Autodesk Fusion 360 part; units mm, degrees
(part 2 of 6)
  spline S14 degree 5 poles (-31.4433, -12.4785) (-31.4662, -12.4876) (-31.5115, -12.5064) (-31.5784, -12.5368) (-31.6657, -12.5814) (-31.7722, -12.6426) (-31.8768, -12.7077) (-31.9803, -12.7753) (-32.0831, -12.8441) (-32.1855, -12.9138) (-32.2874, -12.9845) (-32.3887, -13.0565) (-32.489, -13.1301) (-32.5883, -13.2057) (-32.6866, -13.2831) (-32.7839, -13.3623) (-32.8804, -13.443) (-32.9762, -13.5248) (-33.0713, -13.6077) (-33.1659, -13.6917) (-33.2598, -13.7766) (-33.353, -13.8626) (-33.4455, -13.9498) (-33.5373, -14.0381) (-33.6284, -14.1276) (-33.7188, -14.2182) (-33.8085, -14.3097) (-33.8976, -14.4022) (-33.986, -14.4957) (-34.0738, -14.5901) (-34.161, -14.6853) (-34.2476, -14.7815) (-34.3335, -14.8786) (-34.4188, -14.9765) (-34.5034, -15.0753) (-34.5874, -15.175) (-34.6708, -15.2756) (-34.7536, -15.3769) (-34.8357, -15.4791) (-34.9173, -15.582) (-34.9982, -15.6857) (-35.0785, -15.7902) (-35.1582, -15.8955) (-35.2373, -16.0015) (-35.3158, -16.1083) (-35.3936, -16.2158) (-35.4709, -16.324) (-35.5475, -16.433) (-35.6236, -16.5427) (-35.699, -16.653) (-35.7739, -16.764) (-35.8481, -16.8758) (-35.9218, -16.9882) (-35.9948, -17.1012) (-36.0672, -17.2149) (-36.1391, -17.3293) (-36.2103, -17.4443) (-36.2809, -17.56) (-36.351, -17.6763) (-36.4204, -17.7932) (-36.4892, -17.9107) (-36.5575, -18.0288) (-36.6251, -18.1475) (-36.6921, -18.2669) (-36.7586, -18.3868) (-36.8244, -18.5073) (-36.8897, -18.6283) (-36.9543, -18.75) (-37.0183, -18.8722) (-37.0818, -18.995) (-37.1446, -19.1183) (-37.1944, -19.2174) (-37.2315, -19.292) (-37.2561, -19.3418) (-37.2683, -19.3667) knots 0 0 0 0 0 0 0.01428571 0.02857143 0.04285714 0.05714286 0.07142857 0.08571429 0.1 0.11428571 0.12857143 0.14285714 0.15714286 0.17142857 0.18571429 0.2 0.21428571 0.22857143 0.24285714 0.25714286 0.27142857 0.28571429 0.3 0.31428571 0.32857143 0.34285714 0.35714286 0.37142857 0.38571429 0.4 0.41428571 0.42857143 0.44285714 0.45714286 0.47142857 0.48571429 0.5 0.51428571 0.52857143 0.54285714 0.55714286 0.57142857 0.58571429 0.6 0.61428571 0.62857143 0.64285714 0.65714286 0.67142857 0.68571429 0.7 0.71428571 0.72857143 0.74285714 0.75714286 0.77142857 0.78571429 0.8 0.81428571 0.82857143 0.84285714 0.85714286 0.87142857 0.88571429 0.9 0.91428571 0.92857143 0.94285714 0.95714286 0.97142857 0.98571429 1 1 1 1 1 1
  arc A30 (-37.2683, -19.3667) -> (-35.4063, -22.592) centre (0, 0) ccw
  spline S15 degree 5 poles (-35.4063, -22.592) (-35.3785, -22.5938) (-35.3231, -22.5974) (-35.2399, -22.6026) (-35.1292, -22.609) (-34.991, -22.6163) (-34.853, -22.6227) (-34.7151, -22.6284) (-34.5774, -22.6332) (-34.44, -22.6372) (-34.3027, -22.6405) (-34.1656, -22.6429) (-34.0288, -22.6445) (-33.8921, -22.6453) (-33.7557, -22.6453) (-33.6195, -22.6444) (-33.4836, -22.6427) (-33.3479, -22.6402) (-33.2124, -22.6369) (-33.0772, -22.6327) (-32.9422, -22.6277) (-32.8075, -22.6218) (-32.6731, -22.6151) (-32.5389, -22.6075) (-32.405, -22.5991) (-32.2714, -22.5898) (-32.1382, -22.5796) (-32.0052, -22.5686) (-31.8725, -22.5567) (-31.7401, -22.5439) (-31.6081, -22.5302) (-31.4764, -22.5156) (-31.345, -22.5001) (-31.214, -22.4837) (-31.0833, -22.4664) (-30.9531, -22.4482) (-30.8231, -22.4291) (-30.6936, -22.409) (-30.5644, -22.388) (-30.4357, -22.3661) (-30.3073, -22.3432) (-30.1794, -22.3193) (-30.0519, -22.2944) (-29.9249, -22.2685) (-29.7984, -22.2417) (-29.6723, -22.2138) (-29.5467, -22.1849) (-29.4215, -22.155) (-29.2968, -22.1242) (-29.1727, -22.0922) (-29.0491, -22.0592) (-28.926, -22.0251) (-28.8036, -21.9898) (-28.6819, -21.9532) (-28.5608, -21.9155) (-28.4403, -21.8767) (-28.3203, -21.8367) (-28.2009, -21.7958) (-28.0821, -21.7538) (-27.964, -21.7105) (-27.8468, -21.6658) (-27.7306, -21.6195) (-27.6155, -21.5713) (-27.5016, -21.5212) (-27.3886, -21.4695) (-27.2765, -21.4166) (-27.1649, -21.3627) (-27.0539, -21.3081) (-26.9436, -21.2522) (-26.8349, -21.1942) (-26.7287, -21.1326) (-26.6464, -21.0793) (-26.5866, -21.0365) (-26.5477, -21.0067) (-26.5284, -20.9915) knots -1 -1 -1 -1 -1 -1 -0.98571429 -0.97142857 -0.95714286 -0.94285714 -0.92857143 -0.91428571 -0.9 -0.88571429 -0.87142857 -0.85714286 -0.84285714 -0.82857143 -0.81428571 -0.8 -0.78571429 -0.77142857 -0.75714286 -0.74285714 -0.72857143 -0.71428571 -0.7 -0.68571429 -0.67142857 -0.65714286 -0.64285714 -0.62857143 -0.61428571 -0.6 -0.58571429 -0.57142857 -0.55714286 -0.54285714 -0.52857143 -0.51428571 -0.5 -0.48571429 -0.47142857 -0.45714286 -0.44285714 -0.42857143 -0.41428571 -0.4 -0.38571429 -0.37142857 -0.35714286 -0.34285714 -0.32857143 -0.31428571 -0.3 -0.28571429 -0.27142857 -0.25714286 -0.24285714 -0.22857143 -0.21428571 -0.2 -0.18571429 -0.17142857 -0.15714286 -0.14285714 -0.12857143 -0.11428571 -0.1 -0.08571429 -0.07142857 -0.05714286 -0.04285714 -0.02857143 -0.01428571 0 0 0 0 0 0
  line L15 (-26.5284, -20.9915) -> (-24.3049, -19.232)
  arc A31 (-21.5786, -19.461) -> (-24.3049, -19.232) centre (-23.0639, -20.8004) ccw
  arc A32 (-21.5786, -19.461) -> (-19.461, -21.5786) centre (0, 0) ccw
  arc A33 (-19.232, -24.3049) -> (-19.461, -21.5786) centre (-20.8004, -23.0639) ccw
  line L16 (-19.232, -24.3049) -> (-20.9915, -26.5284)
  spline S16 degree 5 poles (-20.9915, -26.5284) (-21.0067, -26.5477) (-21.0365, -26.5866) (-21.0793, -26.6464) (-21.1326, -26.7287) (-21.1942, -26.8349) (-21.2522, -26.9436) (-21.3081, -27.0539) (-21.3627, -27.1649) (-21.4166, -27.2765) (-21.4695, -27.3886) (-21.5212, -27.5016) (-21.5713, -27.6155) (-21.6195, -27.7306) (-21.6658, -27.8468) (-21.7105, -27.964) (-21.7538, -28.0821) (-21.7958, -28.2009) (-21.8367, -28.3203) (-21.8767, -28.4403) (-21.9155, -28.5608) (-21.9532, -28.6819) (-21.9898, -28.8036) (-22.0251, -28.926) (-22.0592, -29.0491) (-22.0922, -29.1727) (-22.1242, -29.2968) (-22.155, -29.4215) (-22.1849, -29.5467) (-22.2138, -29.6723) (-22.2417, -29.7984) (-22.2685, -29.9249) (-22.2944, -30.0519) (-22.3193, -30.1794) (-22.3432, -30.3073) (-22.3661, -30.4357) (-22.388, -30.5644) (-22.409, -30.6936) (-22.4291, -30.8231) (-22.4482, -30.9531) (-22.4664, -31.0833) (-22.4837, -31.214) (-22.5001, -31.345) (-22.5156, -31.4764) (-22.5302, -31.6081) (-22.5439, -31.7401) (-22.5567, -31.8725) (-22.5686, -32.0052) (-22.5796, -32.1382) (-22.5898, -32.2714) (-22.5991, -32.405) (-22.6075, -32.5389) (-22.6151, -32.6731) (-22.6218, -32.8075) (-22.6277, -32.9422) (-22.6327, -33.0772) (-22.6369, -33.2124) (-22.6402, -33.3479) (-22.6427, -33.4836) (-22.6444, -33.6195) (-22.6453, -33.7557) (-22.6453, -33.8921) (-22.6445, -34.0288) (-22.6429, -34.1656) (-22.6405, -34.3027) (-22.6372, -34.44) (-22.6332, -34.5774) (-22.6284, -34.7151) (-22.6227, -34.853) (-22.6163, -34.991) (-22.609, -35.1292) (-22.6026, -35.2399) (-22.5974, -35.3231) (-22.5938, -35.3785) (-22.592, -35.4063) knots 0 0 0 0 0 0 0.01428571 0.02857143 0.04285714 0.05714286 0.07142857 0.08571429 0.1 0.11428571 0.12857143 0.14285714 0.15714286 0.17142857 0.18571429 0.2 0.21428571 0.22857143 0.24285714 0.25714286 0.27142857 0.28571429 0.3 0.31428571 0.32857143 0.34285714 0.35714286 0.37142857 0.38571429 0.4 0.41428571 0.42857143 0.44285714 0.45714286 0.47142857 0.48571429 0.5 0.51428571 0.52857143 0.54285714 0.55714286 0.57142857 0.58571429 0.6 0.61428571 0.62857143 0.64285714 0.65714286 0.67142857 0.68571429 0.7 0.71428571 0.72857143 0.74285714 0.75714286 0.77142857 0.78571429 0.8 0.81428571 0.82857143 0.84285714 0.85714286 0.87142857 0.88571429 0.9 0.91428571 0.92857143 0.94285714 0.95714286 0.97142857 0.98571429 1 1 1 1 1 1
  arc A34 (-22.592, -35.4063) -> (-19.3667, -37.2683) centre (0, 0) ccw
  spline S17 degree 5 poles (-19.3667, -37.2683) (-19.3418, -37.2561) (-19.292, -37.2315) (-19.2174, -37.1944) (-19.1183, -37.1446) (-18.995, -37.0818) (-18.8722, -37.0183) (-18.75, -36.9543) (-18.6283, -36.8897) (-18.5073, -36.8244) (-18.3868, -36.7586) (-18.2669, -36.6921) (-18.1475, -36.6251) (-18.0288, -36.5575) (-17.9107, -36.4892) (-17.7932, -36.4204) (-17.6763, -36.351) (-17.56, -36.2809) (-17.4443, -36.2103) (-17.3293, -36.1391) (-17.2149, -36.0672) (-17.1012, -35.9948) (-16.9882, -35.9218) (-16.8758, -35.8481) (-16.764, -35.7739) (-16.653, -35.699) (-16.5427, -35.6236) (-16.433, -35.5475) (-16.324, -35.4709) (-16.2158, -35.3936) (-16.1083, -35.3158) (-16.0015, -35.2373) (-15.8955, -35.1582) (-15.7902, -35.0785) (-15.6857, -34.9982) (-15.582, -34.9173) (-15.4791, -34.8357) (-15.3769, -34.7536) (-15.2756, -34.6708) (-15.175, -34.5874) (-15.0753, -34.5034) (-14.9765, -34.4188) (-14.8786, -34.3335) (-14.7815, -34.2476) (-14.6853, -34.161) (-14.5901, -34.0738) (-14.4957, -33.986) (-14.4022, -33.8976) (-14.3097, -33.8085) (-14.2182, -33.7188) (-14.1276, -33.6284) (-14.0381, -33.5373) (-13.9498, -33.4455) (-13.8626, -33.353) (-13.7766, -33.2598) (-13.6917, -33.1659) (-13.6077, -33.0713) (-13.5248, -32.9762) (-13.443, -32.8804) (-13.3623, -32.7839) (-13.2831, -32.6866) (-13.2057, -32.5883) (-13.1301, -32.489) (-13.0565, -32.3887) (-12.9845, -32.2874) (-12.9138, -32.1855) (-12.8441, -32.0831) (-12.7753, -31.9803) (-12.7077, -31.8768) (-12.6426, -31.7722) (-12.5814, -31.6657) (-12.5368, -31.5784) (-12.5064, -31.5115) (-12.4876, -31.4662) (-12.4785, -31.4433) knots -1 -1 -1 -1 -1 -1 -0.98571429 -0.97142857 -0.95714286 -0.94285714 -0.92857143 -0.91428571 -0.9 -0.88571429 -0.87142857 -0.85714286 -0.84285714 -0.82857143 -0.81428571 -0.8 -0.78571429 -0.77142857 -0.75714286 -0.74285714 -0.72857143 -0.71428571 -0.7 -0.68571429 -0.67142857 -0.65714286 -0.64285714 -0.62857143 -0.61428571 -0.6 -0.58571429 -0.57142857 -0.55714286 -0.54285714 -0.52857143 -0.51428571 -0.5 -0.48571429 -0.47142857 -0.45714286 -0.44285714 -0.42857143 -0.41428571 -0.4 -0.38571429 -0.37142857 -0.35714286 -0.34285714 -0.32857143 -0.31428571 -0.3 -0.28571429 -0.27142857 -0.25714286 -0.24285714 -0.22857143 -0.21428571 -0.2 -0.18571429 -0.17142857 -0.15714286 -0.14285714 -0.12857143 -0.11428571 -0.1 -0.08571429 -0.07142857 -0.05714286 -0.04285714 -0.02857143 -0.01428571 0 0 0 0 0 0
  line L17 (-12.4785, -31.4433) -> (-11.4326, -28.8079)
  arc A35 (-8.9572, -27.643) -> (-11.4326, -28.8079) centre (-9.5737, -29.5456) ccw
  arc A36 (-8.9572, -27.643) -> (-6.0644, -28.4181) centre (0, 0) ccw
  arc A37 (-4.503, -30.6647) -> (-6.0644, -28.4181) centre (-6.4818, -30.3741) ccw
  line L18 (-4.503, -30.6647) -> (-4.9149, -33.47)
  spline S18 degree 5 poles (-4.9149, -33.47) (-4.9185, -33.4943) (-4.9249, -33.543) (-4.932, -33.6161) (-4.9371, -33.714) (-4.9373, -33.8368) (-4.9332, -33.96) (-4.9264, -34.0834) (-4.9182, -34.2068) (-4.9091, -34.3304) (-4.8988, -34.454) (-4.8871, -34.5776) (-4.8735, -34.7013) (-4.8577, -34.8251) (-4.8398, -34.949) (-4.8198, -35.0728) (-4.7983, -35.1967) (-4.7752, -35.3206) (-4.751, -35.4445) (-4.7256, -35.5683) (-4.699, -35.6921) (-4.6711, -35.8159) (-4.6419, -35.9396) (-4.6113, -36.0632) (-4.5793, -36.1868) (-4.5461, -36.3104) (-4.5117, -36.4339) (-4.4761, -36.5573) (-4.4394, -36.6806) (-4.4016, -36.8038) (-4.3627, -36.927) (-4.3226, -37.05) (-4.2815, -37.173) (-4.2393, -37.2958) (-4.1961, -37.4185) (-4.1517, -37.5411) (-4.1064, -37.6636) (-4.06, -37.7859) (-4.0126, -37.9082) (-3.9642, -38.0302) (-3.9148, -38.1522) (-3.8645, -38.274) (-3.8132, -38.3956) (-3.7609, -38.5172) (-3.7077, -38.6385) (-3.6535, -38.7597) (-3.5984, -38.8807) (-3.5424, -39.0016) (-3.4854, -39.1223) (-3.4276, -39.2428) (-3.3689, -39.3631) (-3.3092, -39.4833) (-3.2487, -39.6032) (-3.1873, -39.723) (-3.125, -39.8426) (-3.0619, -39.962) (-2.9979, -40.0812) (-2.9331, -40.2002) (-2.8674, -40.319) (-2.8009, -40.4376) (-2.7335, -40.5559) (-2.6653, -40.6741) (-2.5963, -40.792) (-2.5265, -40.9098) (-2.4559, -41.0273) (-2.3844, -41.1445) (-2.3122, -41.2616) (-2.2392, -41.3783) (-2.1654, -41.4949) (-2.0908, -41.6112) (-2.0154, -41.7273) (-1.9545, -41.82) (-1.9084, -41.8894) (-1.8776, -41.9356) (-1.8621, -41.9587) knots 0 0 0 0 0 0 0.01428571 0.02857143 0.04285714 0.05714286 0.07142857 0.08571429 0.1 0.11428571 0.12857143 0.14285714 0.15714286 0.17142857 0.18571429 0.2 0.21428571 0.22857143 0.24285714 0.25714286 0.27142857 0.28571429 0.3 0.31428571 0.32857143 0.34285714 0.35714286 0.37142857 0.38571429 0.4 0.41428571 0.42857143 0.44285714 0.45714286 0.47142857 0.48571429 0.5 0.51428571 0.52857143 0.54285714 0.55714286 0.57142857 0.58571429 0.6 0.61428571 0.62857143 0.64285714 0.65714286 0.67142857 0.68571429 0.7 0.71428571 0.72857143 0.74285714 0.75714286 0.77142857 0.78571429 0.8 0.81428571 0.82857143 0.84285714 0.85714286 0.87142857 0.88571429 0.9 0.91428571 0.92857143 0.94285714 0.95714286 0.97142857 0.98571429 1 1 1 1 1 1
  arc A38 (-1.8621, -41.9587) -> (1.8621, -41.9587) centre (0, 0) ccw
  spline S19 degree 5 poles (1.8621, -41.9587) (1.8776, -41.9356) (1.9084, -41.8894) (1.9545, -41.82) (2.0154, -41.7273) (2.0908, -41.6112) (2.1654, -41.4949) (2.2392, -41.3783) (2.3122, -41.2616) (2.3844, -41.1445) (2.4559, -41.0273) (2.5265, -40.9098) (2.5963, -40.792) (2.6653, -40.6741) (2.7335, -40.5559) (2.8009, -40.4376) (2.8674, -40.319) (2.9331, -40.2002) (2.9979, -40.0812) (3.0619, -39.962) (3.125, -39.8426) (3.1873, -39.723) (3.2487, -39.6032) (3.3092, -39.4833) (3.3689, -39.3631) (3.4276, -39.2428) (3.4854, -39.1223) (3.5424, -39.0016) (3.5984, -38.8807) (3.6535, -38.7597) (3.7077, -38.6385) (3.7609, -38.5172) (3.8132, -38.3956) (3.8645, -38.274) (3.9148, -38.1522) (3.9642, -38.0302) (4.0126, -37.9082) (4.06, -37.7859) (4.1064, -37.6636) (4.1517, -37.5411) (4.1961, -37.4185) (4.2393, -37.2958) (4.2815, -37.173) (4.3226, -37.05) (4.3627, -36.927) (4.4016, -36.8038) (4.4394, -36.6806) (4.4761, -36.5573) (4.5117, -36.4339) (4.5461, -36.3104) (4.5793, -36.1868) (4.6113, -36.0632) (4.6419, -35.9396) (4.6711, -35.8159) (4.699, -35.6921) (4.7256, -35.5683) (4.751, -35.4445) (4.7752, -35.3206) (4.7983, -35.1967) (4.8198, -35.0728) (4.8398, -34.949) (4.8577, -34.8251) (4.8735, -34.7013) (4.8871, -34.5776) (4.8988, -34.454) (4.9091, -34.3304) (4.9182, -34.2068) (4.9264, -34.0834) (4.9332, -33.96) (4.9373, -33.8368) (4.9371, -33.714) (4.932, -33.6161) (4.9249, -33.543) (4.9185, -33.4943) (4.9149, -33.47) knots -1 -1 -1 -1 -1 -1 -0.98571429 -0.97142857 -0.95714286 -0.94285714 -0.92857143 -0.91428571 -0.9 -0.88571429 -0.87142857 -0.85714286 -0.84285714 -0.82857143 -0.81428571 -0.8 -0.78571429 -0.77142857 -0.75714286 -0.74285714 -0.72857143 -0.71428571 -0.7 -0.68571429 -0.67142857 -0.65714286 -0.64285714 -0.62857143 -0.61428571 -0.6 -0.58571429 -0.57142857 -0.55714286 -0.54285714 -0.52857143 -0.51428571 -0.5 -0.48571429 -0.47142857 -0.45714286 -0.44285714 -0.42857143 -0.41428571 -0.4 -0.38571429 -0.37142857 -0.35714286 -0.34285714 -0.32857143 -0.31428571 -0.3 -0.28571429 -0.27142857 -0.25714286 -0.24285714 -0.22857143 -0.21428571 -0.2 -0.18571429 -0.17142857 -0.15714286 -0.14285714 -0.12857143 -0.11428571 -0.1 -0.08571429 -0.07142857 -0.05714286 -0.04285714 -0.02857143 -0.01428571 0 0 0 0 0 0
  line L19 (4.9149, -33.47) -> (4.503, -30.6647)
  arc A39 (6.0644, -28.4181) -> (4.503, -30.6647) centre (6.4818, -30.3741) ccw
  arc A40 (6.0644, -28.4181) -> (8.9572, -27.643) centre (0, 0) ccw
  arc A41 (11.4326, -28.8079) -> (8.9572, -27.643) centre (9.5737, -29.5456) ccw
  line L20 (11.4326, -28.8079) -> (12.4785, -31.4433)
  spline S20 degree 5 poles (12.4785, -31.4433) (12.4876, -31.4662) (12.5064, -31.5115) (12.5368, -31.5784) (12.5814, -31.6657) (12.6426, -31.7722) (12.7077, -31.8768) (12.7753, -31.9803) (12.8441, -32.0831) (12.9138, -32.1855) (12.9845, -32.2874) (13.0565, -32.3887) (13.1301, -32.489) (13.2057, -32.5883) (13.2831, -32.6866) (13.3623, -32.7839) (13.443, -32.8804) (13.5248, -32.9762) (13.6077, -33.0713) (13.6917, -33.1659) (13.7766, -33.2598) (13.8626, -33.353) (13.9498, -33.4455) (14.0381, -33.5373) (14.1276, -33.6284) (14.2182, -33.7188) (14.3097, -33.8085) (14.4022, -33.8976) (14.4957, -33.986) (14.5901, -34.0738) (14.6853, -34.161) (14.7815, -34.2476) (14.8786, -34.3335) (14.9765, -34.4188) (15.0753, -34.5034) (15.175, -34.5874) (15.2756, -34.6708) (15.3769, -34.7536) (15.4791, -34.8357) (15.582, -34.9173) (15.6857, -34.9982) (15.7902, -35.0785) (15.8955, -35.1582) (16.0015, -35.2373) (16.1083, -35.3158) (16.2158, -35.3936) (16.324, -35.4709) (16.433, -35.5475) (16.5427, -35.6236) (16.653, -35.699) (16.764, -35.7739) (16.8758, -35.8481) (16.9882, -35.9218) (17.1012, -35.9948) (17.2149, -36.0672) (17.3293, -36.1391) (17.4443, -36.2103) (17.56, -36.2809) (17.6763, -36.351) (17.7932, -36.4204) (17.9107, -36.4892) (18.0288, -36.5575) (18.1475, -36.6251) (18.2669, -36.6921) (18.3868, -36.7586) (18.5073, -36.8244) (18.6283, -36.8897) (18.75, -36.9543) (18.8722, -37.0183) (18.995, -37.0818) (19.1183, -37.1446) (19.2174, -37.1944) (19.292, -37.2315) (19.3418, -37.2561) (19.3667, -37.2683) knots 0 0 0 0 0 0 0.01428571 0.02857143 0.04285714 0.05714286 0.07142857 0.08571429 0.1 0.11428571 0.12857143 0.14285714 0.15714286 0.17142857 0.18571429 0.2 0.21428571 0.22857143 0.24285714 0.25714286 0.27142857 0.28571429 0.3 0.31428571 0.32857143 0.34285714 0.35714286 0.37142857 0.38571429 0.4 0.41428571 0.42857143 0.44285714 0.45714286 0.47142857 0.48571429 0.5 0.51428571 0.52857143 0.54285714 0.55714286 0.57142857 0.58571429 0.6 0.61428571 0.62857143 0.64285714 0.65714286 0.67142857 0.68571429 0.7 0.71428571 0.72857143 0.74285714 0.75714286 0.77142857 0.78571429 0.8 0.81428571 0.82857143 0.84285714 0.85714286 0.87142857 0.88571429 0.9 0.91428571 0.92857143 0.94285714 0.95714286 0.97142857 0.98571429 1 1 1 1 1 1
  arc A42 (19.3667, -37.2683) -> (22.592, -35.4063) centre (0, 0) ccw
  spline S21 degree 5 poles (22.592, -35.4063) (22.5938, -35.3785) (22.5974, -35.3231) (22.6026, -35.2399) (22.609, -35.1292) (22.6163, -34.991) (22.6227, -34.853) (22.6284, -34.7151) (22.6332, -34.5774) (22.6372, -34.44) (22.6405, -34.3027) (22.6429, -34.1656) (22.6445, -34.0288) (22.6453, -33.8921) (22.6453, -33.7557) (22.6444, -33.6195) (22.6427, -33.4836) (22.6402, -33.3479) (22.6369, -33.2124) (22.6327, -33.0772) (22.6277, -32.9422) (22.6218, -32.8075) (22.6151, -32.6731) (22.6075, -32.5389) (22.5991, -32.405) (22.5898, -32.2714) (22.5796, -32.1382) (22.5686, -32.0052) (22.5567, -31.8725) (22.5439, -31.7401) (22.5302, -31.6081) (22.5156, -31.4764) (22.5001, -31.345) (22.4837, -31.214) (22.4664, -31.0833) (22.4482, -30.9531) (22.4291, -30.8231) (22.409, -30.6936) (22.388, -30.5644) (22.3661, -30.4357) (22.3432, -30.3073) (22.3193, -30.1794) (22.2944, -30.0519) (22.2685, -29.9249) (22.2417, -29.7984) (22.2138, -29.6723) (22.1849, -29.5467) (22.155, -29.4215) (22.1242, -29.2968) (22.0922, -29.1727) (22.0592, -29.0491) (22.0251, -28.926) (21.9898, -28.8036) (21.9532, -28.6819) (21.9155, -28.5608) (21.8767, -28.4403) (21.8367, -28.3203) (21.7958, -28.2009) (21.7538, -28.0821) (21.7105, -27.964) (21.6658, -27.8468) (21.6195, -27.7306) (21.5713, -27.6155) (21.5212, -27.5016) (21.4695, -27.3886) (21.4166, -27.2765) (21.3627, -27.1649) (21.3081, -27.0539) (21.2522, -26.9436) (21.1942, -26.8349) (21.1326, -26.7287) (21.0793, -26.6464) (21.0365, -26.5866) (21.0067, -26.5477) (20.9915, -26.5284) knots -1 -1 -1 -1 -1 -1 -0.98571429 -0.97142857 -0.95714286 -0.94285714 -0.92857143 -0.91428571 -0.9 -0.88571429 -0.87142857 -0.85714286 -0.84285714 -0.82857143 -0.81428571 -0.8 -0.78571429 -0.77142857 -0.75714286 -0.74285714 -0.72857143 -0.71428571 -0.7 -0.68571429 -0.67142857 -0.65714286 -0.64285714 -0.62857143 -0.61428571 -0.6 -0.58571429 -0.57142857 -0.55714286 -0.54285714 -0.52857143 -0.51428571 -0.5 -0.48571429 -0.47142857 -0.45714286 -0.44285714 -0.42857143 -0.41428571 -0.4 -0.38571429 -0.37142857 -0.35714286 -0.34285714 -0.32857143 -0.31428571 -0.3 -0.28571429 -0.27142857 -0.25714286 -0.24285714 -0.22857143 -0.21428571 -0.2 -0.18571429 -0.17142857 -0.15714286 -0.14285714 -0.12857143 -0.11428571 -0.1 -0.08571429 -0.07142857 -0.05714286 -0.04285714 -0.02857143 -0.01428571 0 0 0 0 0 0
  line L21 (20.9915, -26.5284) -> (19.232, -24.3049)
  arc A43 (19.461, -21.5786) -> (19.232, -24.3049) centre (20.8004, -23.0639) ccw
  arc A44 (19.461, -21.5786) -> (21.5786, -19.461) centre (0, 0) ccw
  arc A45 (24.3049, -19.232) -> (21.5786, -19.461) centre (23.0639, -20.8004) ccw
  line L22 (24.3049, -19.232) -> (26.5284, -20.9915)
  spline S22 degree 5 poles (26.5284, -20.9915) (26.5477, -21.0067) (26.5866, -21.0365) (26.6464, -21.0793) (26.7287, -21.1326) (26.8349, -21.1942) (26.9436, -21.2522) (27.0539, -21.3081) (27.1649, -21.3627) (27.2765, -21.4166) (27.3886, -21.4695) (27.5016, -21.5212) (27.6155, -21.5713) (27.7306, -21.6195) (27.8468, -21.6658) (27.964, -21.7105) (28.0821, -21.7538) (28.2009, -21.7958) (28.3203, -21.8367) (28.4403, -21.8767) (28.5608, -21.9155) (28.6819, -21.9532) (28.8036, -21.9898) (28.926, -22.0251) (29.0491, -22.0592) (29.1727, -22.0922) (29.2968, -22.1242) (29.4215, -22.155) (29.5467, -22.1849) (29.6723, -22.2138) (29.7984, -22.2417) (29.9249, -22.2685) (30.0519, -22.2944) (30.1794, -22.3193) (30.3073, -22.3432) (30.4357, -22.3661) (30.5644, -22.388) (30.6936, -22.409) (30.8231, -22.4291) (30.9531, -22.4482) (31.0833, -22.4664) (31.214, -22.4837) (31.345, -22.5001) (31.4764, -22.5156) (31.6081, -22.5302) (31.7401, -22.5439) (31.8725, -22.5567) (32.0052, -22.5686) (32.1382, -22.5796) (32.2714, -22.5898) (32.405, -22.5991) (32.5389, -22.6075) (32.6731, -22.6151) (32.8075, -22.6218) (32.9422, -22.6277) (33.0772, -22.6327) (33.2124, -22.6369) (33.3479, -22.6402) (33.4836, -22.6427) (33.6195, -22.6444) (33.7557, -22.6453) (33.8921, -22.6453) (34.0288, -22.6445) (34.1656, -22.6429) (34.3027, -22.6405) (34.44, -22.6372) (34.5774, -22.6332) (34.7151, -22.6284) (34.853, -22.6227) (34.991, -22.6163) (35.1292, -22.609) (35.2399, -22.6026) (35.3231, -22.5974) (35.3785, -22.5938) (35.4063, -22.592) knots 0 0 0 0 0 0 0.01428571 0.02857143 0.04285714 0.05714286 0.07142857 0.08571429 0.1 0.11428571 0.12857143 0.14285714 0.15714286 0.17142857 0.18571429 0.2 0.21428571 0.22857143 0.24285714 0.25714286 0.27142857 0.28571429 0.3 0.31428571 0.32857143 0.34285714 0.35714286 0.37142857 0.38571429 0.4 0.41428571 0.42857143 0.44285714 0.45714286 0.47142857 0.48571429 0.5 0.51428571 0.52857143 0.54285714 0.55714286 0.57142857 0.58571429 0.6 0.61428571 0.62857143 0.64285714 0.65714286 0.67142857 0.68571429 0.7 0.71428571 0.72857143 0.74285714 0.75714286 0.77142857 0.78571429 0.8 0.81428571 0.82857143 0.84285714 0.85714286 0.87142857 0.88571429 0.9 0.91428571 0.92857143 0.94285714 0.95714286 0.97142857 0.98571429 1 1 1 1 1 1
  arc A46 (35.4063, -22.592) -> (37.2683, -19.3667) centre (0, 0) ccw
  spline S23 degree 5 poles (37.2683, -19.3667) (37.2561, -19.3418) (37.2315, -19.292) (37.1944, -19.2174) (37.1446, -19.1183) (37.0818, -18.995) (37.0183, -18.8722) (36.9543, -18.75) (36.8897, -18.6283) (36.8244, -18.5073) (36.7586, -18.3868) (36.6921, -18.2669) (36.6251, -18.1475) (36.5575, -18.0288) (36.4892, -17.9107) (36.4204, -17.7932) (36.351, -17.6763) (36.2809, -17.56) (36.2103, -17.4443) (36.1391, -17.3293) (36.0672, -17.2149) (35.9948, -17.1012) (35.9218, -16.9882) (35.8481, -16.8758) (35.7739, -16.764) (35.699, -16.653) (35.6236, -16.5427) (35.5475, -16.433) (35.4709, -16.324) (35.3936, -16.2158) (35.3158, -16.1083) (35.2373, -16.0015) (35.1582, -15.8955) (35.0785, -15.7902) (34.9982, -15.6857) (34.9173, -15.582) (34.8357, -15.4791) (34.7536, -15.3769) (34.6708, -15.2756) (34.5874, -15.175) (34.5034, -15.0753) (34.4188, -14.9765) (34.3335, -14.8786) (34.2476, -14.7815) (34.161, -14.6853) (34.0738, -14.5901) (33.986, -14.4957) (33.8976, -14.4022) (33.8085, -14.3097) (33.7188, -14.2182) (33.6284, -14.1276) (33.5373, -14.0381) (33.4455, -13.9498) (33.353, -13.8626) (33.2598, -13.7766) (33.1659, -13.6917) (33.0713, -13.6077) (32.9762, -13.5248) (32.8804, -13.443) (32.7839, -13.3623) (32.6866, -13.2831) (32.5883, -13.2057) (32.489, -13.1301) (32.3887, -13.0565) (32.2874, -12.9845) (32.1855, -12.9138) (32.0831, -12.8441) (31.9803, -12.7753) (31.8768, -12.7077) (31.7722, -12.6426) (31.6657, -12.5814) (31.5784, -12.5368) (31.5115, -12.5064) (31.4662, -12.4876) (31.4433, -12.4785) knots -1 -1 -1 -1 -1 -1 -0.98571429 -0.97142857 -0.95714286 -0.94285714 -0.92857143 -0.91428571 -0.9 -0.88571429 -0.87142857 -0.85714286 -0.84285714 -0.82857143 -0.81428571 -0.8 -0.78571429 -0.77142857 -0.75714286 -0.74285714 -0.72857143 -0.71428571 -0.7 -0.68571429 -0.67142857 -0.65714286 -0.64285714 -0.62857143 -0.61428571 -0.6 -0.58571429 -0.57142857 -0.55714286 -0.54285714 -0.52857143 -0.51428571 -0.5 -0.48571429 -0.47142857 -0.45714286 -0.44285714 -0.42857143 -0.41428571 -0.4 -0.38571429 -0.37142857 -0.35714286 -0.34285714 -0.32857143 -0.31428571 -0.3 -0.28571429 -0.27142857 -0.25714286 -0.24285714 -0.22857143 -0.21428571 -0.2 -0.18571429 -0.17142857 -0.15714286 -0.14285714 -0.12857143 -0.11428571 -0.1 -0.08571429 -0.07142857 -0.05714286 -0.04285714 -0.02857143 -0.01428571 0 0 0 0 0 0
  line L23 (31.4433, -12.4785) -> (28.8079, -11.4326)
  arc A47 (27.643, -8.9572) -> (28.8079, -11.4326) centre (29.5456, -9.5737) ccw
  circle A48 centre (0, 0) radius 2.5
  arc A49 (173.4789, -18.1364) -> (174.1765, -15.5329) centre (111, 0) ccw
  arc A50 (176.538, -14.0549) -> (174.1765, -15.5329) centre (176.1187, -16.0104) ccw
  line L24 (176.538, -14.0549) -> (177.1537, -14.1869)
  spline S24 degree 5 poles (177.1537, -14.1869) (177.1836, -14.1933) (177.2435, -14.2054) (177.3338, -14.2212) (177.4547, -14.2379) (177.6068, -14.2529) (177.7596, -14.2636) (177.9128, -14.2716) (178.0662, -14.2783) (178.2197, -14.284) (178.3734, -14.2887) (178.5272, -14.2921) (178.6813, -14.2937) (178.8356, -14.2932) (178.9902, -14.2907) (179.145, -14.2862) (179.2999, -14.2801) (179.455, -14.2726) (179.6102, -14.2639) (179.7655, -14.2541) (179.9208, -14.2432) (180.0763, -14.231) (180.2318, -14.2177) (180.3875, -14.203) (180.5432, -14.187) (180.699, -14.1699) (180.8549, -14.1515) (181.0108, -14.1321) (181.1668, -14.1116) (181.3228, -14.0901) (181.4789, -14.0675) (181.635, -14.0439) (181.7911, -14.0193) (181.9473, -13.9936) (182.1034, -13.9669) (182.2596, -13.9393) (182.4159, -13.9106) (182.5721, -13.881) (182.7284, -13.8504) (182.8846, -13.8189) (183.0409, -13.7865) (183.1971, -13.7532) (183.3533, -13.7189) (183.5096, -13.6838) (183.6658, -13.6477) (183.822, -13.6108) (183.9782, -13.573) (184.1343, -13.5344) (184.2905, -13.4948) (184.4466, -13.4545) (184.6026, -13.4132) (184.7587, -13.3712) (184.9147, -13.3283) (185.0707, -13.2846) (185.2266, -13.2401) (185.3825, -13.1947) (185.5383, -13.1486) (185.6941, -13.1017) (185.8498, -13.0539) (186.0055, -13.0054) (186.1611, -12.9561) (186.3167, -12.9061) (186.4722, -12.8552) (186.6276, -12.8036) (186.783, -12.7512) (186.9383, -12.6981) (187.0935, -12.6442) (187.2487, -12.5896) (187.4037, -12.5342) (187.5587, -12.4781) (187.7137, -12.4213) (187.8375, -12.3752) (187.9304, -12.3403) (187.9923, -12.3169) (188.0233, -12.3052) knots 0 0 0 0 0 0 0.01428571 0.02857143 0.04285714 0.05714286 0.07142857 0.08571429 0.1 0.11428571 0.12857143 0.14285714 0.15714286 0.17142857 0.18571429 0.2 0.21428571 0.22857143 0.24285714 0.25714286 0.27142857 0.28571429 0.3 0.31428571 0.32857143 0.34285714 0.35714286 0.37142857 0.38571429 0.4 0.41428571 0.42857143 0.44285714 0.45714286 0.47142857 0.48571429 0.5 0.51428571 0.52857143 0.54285714 0.55714286 0.57142857 0.58571429 0.6 0.61428571 0.62857143 0.64285714 0.65714286 0.67142857 0.68571429 0.7 0.71428571 0.72857143 0.74285714 0.75714286 0.77142857 0.78571429 0.8 0.81428571 0.82857143 0.84285714 0.85714286 0.87142857 0.88571429 0.9 0.91428571 0.92857143 0.94285714 0.95714286 0.97142857 0.98571429 1 1 1 1 1 1
  arc A51 (188.0233, -12.3052) -> (188.5836, -8.0492) centre (111, 0) ccw
  spline S25 degree 5 poles (188.5836, -8.0492) (188.5567, -8.0298) (188.503, -7.9912) (188.4223, -7.9335) (188.3146, -7.8569) (188.1796, -7.7619) (188.0444, -7.6676) (187.909, -7.574) (187.7732, -7.4811) (187.6373, -7.3889) (187.501, -7.2973) (187.3645, -7.2065) (187.2277, -7.1165) (187.0906, -7.0271) (186.9533, -6.9385) (186.8158, -6.8506) (186.678, -6.7634) (186.5399, -6.677) (186.4016, -6.5913) (186.263, -6.5065) (186.1242, -6.4223) (185.9851, -6.339) (185.8457, -6.2564) (185.7061, -6.1746) (185.5663, -6.0936) (185.4262, -6.0134) (185.2859, -5.934) (185.1453, -5.8554) (185.0045, -5.7776) (184.8634, -5.7007) (184.7221, -5.6246) (184.5805, -5.5493) (184.4387, -5.4749) (184.2966, -5.4014) (184.1543, -5.3288) (184.0118, -5.257) (183.869, -5.1862) (183.726, -5.1162) (183.5828, -5.0472) (183.4393, -4.9791) (183.2956, -4.9119) (183.1516, -4.8457) (183.0074, -4.7805) (182.863, -4.7163) (182.7183, -4.6531) (182.5734, -4.5909) (182.4283, -4.5297) (182.2829, -4.4696) (182.1373, -4.4104) (181.9915, -4.3524) (181.8454, -4.2955) (181.6991, -4.2398) (181.5526, -4.1853) (181.4058, -4.1321) (181.2588, -4.0802) (181.1116, -4.0294) (180.9641, -3.9798) (180.8165, -3.9312) (180.6686, -3.8838) (180.5205, -3.8378) (180.3722, -3.7934) (180.2235, -3.751) (180.0746, -3.7106) (179.9254, -3.6722) (179.7759, -3.6356) (179.6262, -3.6004) (179.4764, -3.5662) (179.3265, -3.533) (179.1765, -3.5011) (179.0261, -3.4719) (178.8753, -3.447) (178.7542, -3.4318) (178.663, -3.4237) (178.602, -3.4199) (178.5715, -3.4183) knots -1 -1 -1 -1 -1 -1 -0.98571429 -0.97142857 -0.95714286 -0.94285714 -0.92857143 -0.91428571 -0.9 -0.88571429 -0.87142857 -0.85714286 -0.84285714 -0.82857143 -0.81428571 -0.8 -0.78571429 -0.77142857 -0.75714286 -0.74285714 -0.72857143 -0.71428571 -0.7 -0.68571429 -0.67142857 -0.65714286 -0.64285714 -0.62857143 -0.61428571 -0.6 -0.58571429 -0.57142857 -0.55714286 -0.54285714 -0.52857143 -0.51428571 -0.5 -0.48571429 -0.47142857 -0.45714286 -0.44285714 -0.42857143 -0.41428571 -0.4 -0.38571429 -0.37142857 -0.35714286 -0.34285714 -0.32857143 -0.31428571 -0.3 -0.28571429 -0.27142857 -0.25714286 -0.24285714 -0.22857143 -0.21428571 -0.2 -0.18571429 -0.17142857 -0.15714286 -0.14285714 -0.12857143 -0.11428571 -0.1 -0.08571429 -0.07142857 -0.05714286 -0.04285714 -0.02857143 -0.01428571 0 0 0 0 0 0
  line L25 (178.5715, -3.4183) -> (177.9426, -3.3865)
  arc A52 (176.044, -1.3477) -> (177.9426, -3.3865) centre (178.0436, -1.3891) ccw
  arc A53 (176.044, -1.3477) -> (176.044, 1.3477) centre (111, 0) ccw
  arc A54 (177.9426, 3.3865) -> (176.044, 1.3477) centre (178.0436, 1.3891) ccw
  line L26 (177.9426, 3.3865) -> (178.5715, 3.4183)
  spline S26 degree 5 poles (178.5715, 3.4183) (178.602, 3.4199) (178.663, 3.4237) (178.7542, 3.4318) (178.8753, 3.447) (179.0261, 3.4719) (179.1765, 3.5011) (179.3265, 3.533) (179.4764, 3.5662) (179.6262, 3.6004) (179.7759, 3.6356) (179.9254, 3.6722) (180.0746, 3.7106) (180.2235, 3.751) (180.3722, 3.7934) (180.5205, 3.8378) (180.6686, 3.8838) (180.8165, 3.9312) (180.9641, 3.9798) (181.1116, 4.0294) (181.2588, 4.0802) (181.4058, 4.1321) (181.5526, 4.1853) (181.6991, 4.2398) (181.8454, 4.2955) (181.9915, 4.3524) (182.1373, 4.4104) (182.2829, 4.4696) (182.4283, 4.5297) (182.5734, 4.5909) (182.7183, 4.6531) (182.863, 4.7163) (183.0074, 4.7805) (183.1516, 4.8457) (183.2956, 4.9119) (183.4393, 4.9791) (183.5828, 5.0472) (183.726, 5.1162) (183.869, 5.1862) (184.0118, 5.257) (184.1543, 5.3288) (184.2966, 5.4014) (184.4387, 5.4749) (184.5805, 5.5493) (184.7221, 5.6246) (184.8634, 5.7007) (185.0045, 5.7776) (185.1453, 5.8554) (185.2859, 5.934) (185.4262, 6.0134) (185.5663, 6.0936) (185.7061, 6.1746) (185.8457, 6.2564) (185.9851, 6.339) (186.1242, 6.4223) (186.263, 6.5065) (186.4016, 6.5913) (186.5399, 6.677) (186.678, 6.7634) (186.8158, 6.8506) (186.9533, 6.9385) (187.0906, 7.0271) (187.2277, 7.1165) (187.3645, 7.2065) (187.501, 7.2973) (187.6373, 7.3889) (187.7732, 7.4811) (187.909, 7.574) (188.0444, 7.6676) (188.1796, 7.7619) (188.3146, 7.8569) (188.4223, 7.9335) (188.503, 7.9912) (188.5567, 8.0298) (188.5836, 8.0492) knots 0 0 0 0 0 0 0.01428571 0.02857143 0.04285714 0.05714286 0.07142857 0.08571429 0.1 0.11428571 0.12857143 0.14285714 0.15714286 0.17142857 0.18571429 0.2 0.21428571 0.22857143 0.24285714 0.25714286 0.27142857 0.28571429 0.3 0.31428571 0.32857143 0.34285714 0.35714286 0.37142857 0.38571429 0.4 0.41428571 0.42857143 0.44285714 0.45714286 0.47142857 0.48571429 0.5 0.51428571 0.52857143 0.54285714 0.55714286 0.57142857 0.58571429 0.6 0.61428571 0.62857143 0.64285714 0.65714286 0.67142857 0.68571429 0.7 0.71428571 0.72857143 0.74285714 0.75714286 0.77142857 0.78571429 0.8 0.81428571 0.82857143 0.84285714 0.85714286 0.87142857 0.88571429 0.9 0.91428571 0.92857143 0.94285714 0.95714286 0.97142857 0.98571429 1 1 1 1 1 1
  arc A55 (188.5836, 8.0492) -> (188.0233, 12.3052) centre (111, 0) ccw
  spline S27 degree 5 poles (188.0233, 12.3052) (187.9923, 12.3169) (187.9304, 12.3403) (187.8375, 12.3752) (187.7137, 12.4213) (187.5587, 12.4781) (187.4037, 12.5342) (187.2487, 12.5896) (187.0935, 12.6442) (186.9383, 12.6981) (186.783, 12.7512) (186.6276, 12.8036) (186.4722, 12.8552) (186.3167, 12.9061) (186.1611, 12.9561) (186.0055, 13.0054) (185.8498, 13.0539) (185.6941, 13.1017) (185.5383, 13.1486) (185.3825, 13.1947) (185.2266, 13.2401) (185.0707, 13.2846) (184.9147, 13.3283) (184.7587, 13.3712) (184.6026, 13.4132) (184.4466, 13.4545) (184.2905, 13.4948) (184.1343, 13.5344) (183.9782, 13.573) (183.822, 13.6108) (183.6658, 13.6477) (183.5096, 13.6838) (183.3533, 13.7189) (183.1971, 13.7532) (183.0409, 13.7865) (182.8846, 13.8189) (182.7284, 13.8504) (182.5721, 13.881) (182.4159, 13.9106) (182.2596, 13.9393) (182.1034, 13.9669) (181.9473, 13.9936) (181.7911, 14.0193) (181.635, 14.0439) (181.4789, 14.0675) (181.3228, 14.0901) (181.1668, 14.1116) (181.0108, 14.1321) (180.8549, 14.1515) (180.699, 14.1699) (180.5432, 14.187) (180.3875, 14.203) (180.2318, 14.2177) (180.0763, 14.231) (179.9208, 14.2432) (179.7655, 14.2541) (179.6102, 14.2639) (179.455, 14.2726) (179.2999, 14.2801) (179.145, 14.2862) (178.9902, 14.2907) (178.8356, 14.2932) (178.6813, 14.2937) (178.5272, 14.2921) (178.3734, 14.2887) (178.2197, 14.284) (178.0662, 14.2783) (177.9128, 14.2716) (177.7596, 14.2636) (177.6068, 14.2529) (177.4547, 14.2379) (177.3338, 14.2212) (177.2435, 14.2054) (177.1836, 14.1933) (177.1537, 14.1869) knots -1 -1 -1 -1 -1 -1 -0.98571429 -0.97142857 -0.95714286 -0.94285714 -0.92857143 -0.91428571 -0.9 -0.88571429 -0.87142857 -0.85714286 -0.84285714 -0.82857143 -0.81428571 -0.8 -0.78571429 -0.77142857 -0.75714286 -0.74285714 -0.72857143 -0.71428571 -0.7 -0.68571429 -0.67142857 -0.65714286 -0.64285714 -0.62857143 -0.61428571 -0.6 -0.58571429 -0.57142857 -0.55714286 -0.54285714 -0.52857143 -0.51428571 -0.5 -0.48571429 -0.47142857 -0.45714286 -0.44285714 -0.42857143 -0.41428571 -0.4 -0.38571429 -0.37142857 -0.35714286 -0.34285714 -0.32857143 -0.31428571 -0.3 -0.28571429 -0.27142857 -0.25714286 -0.24285714 -0.22857143 -0.21428571 -0.2 -0.18571429 -0.17142857 -0.15714286 -0.14285714 -0.12857143 -0.11428571 -0.1 -0.08571429 -0.07142857 -0.05714286 -0.04285714 -0.02857143 -0.01428571 0 0 0 0 0 0
  line L27 (177.1537, 14.1869) -> (176.538, 14.0549)
  arc A56 (174.1765, 15.5329) -> (176.538, 14.0549) centre (176.1187, 16.0104) ccw
  arc A57 (174.1765, 15.5329) -> (173.4789, 18.1364) centre (111, 0) ccw
  arc A58 (174.7851, 20.5971) -> (173.4789, 18.1364) centre (175.3996, 18.6939) ccw
  line L28 (174.7851, 20.5971) -> (175.3843, 20.7906)
  spline S28 degree 5 poles (175.3843, 20.7906) (175.4134, 20.8) (175.4713, 20.8195) (175.5573, 20.851) (175.6704, 20.897) (175.8096, 20.9601) (175.9473, 21.0272) (176.084, 21.0968) (176.2202, 21.1677) (176.356, 21.2395) (176.4914, 21.3123) (176.6264, 21.3863) (176.7606, 21.4619) (176.894, 21.5395) (177.0266, 21.619) (177.1584, 21.7003) (177.2895, 21.7831) (177.4201, 21.8671) (177.5501, 21.9522) (177.6797, 22.0383) (177.8088, 22.1255) (177.9373, 22.2137) (178.0653, 22.3031) (178.1928, 22.3936) (178.3197, 22.4853) (178.446, 22.578) (178.5719, 22.6718) (178.6972, 22.7666) (178.822, 22.8624) (178.9464, 22.959) (179.0702, 23.0566) (179.1936, 23.1551) (179.3165, 23.2545) (179.4389, 23.3548) (179.5608, 23.456) (179.6823, 23.5581) (179.8033, 23.661) (179.9238, 23.7648) (180.0438, 23.8694) (180.1634, 23.9748) (180.2825, 24.081) (180.4011, 24.1879) (180.5193, 24.2957) (180.637, 24.4043) (180.7543, 24.5136) (180.8711, 24.6237) (180.9875, 24.7345) (181.1034, 24.8461) (181.2188, 24.9584) (181.3338, 25.0714) (181.4484, 25.1851) (181.5625, 25.2996) (181.6762, 25.4147) (181.7894, 25.5305) (181.9021, 25.647) (182.0145, 25.7642) (182.1264, 25.8821) (182.2378, 26.0007) (182.3488, 26.1199) (182.4594, 26.2397) (182.5695, 26.3602) (182.6792, 26.4814) (182.7884, 26.6031) (182.8972, 26.7256) (183.0056, 26.8486) (183.1135, 26.9723) (183.221, 27.0965) (183.3281, 27.2214) (183.4347, 27.3469) (183.5409, 27.473) (183.6466, 27.5997) (183.7309, 27.7015) (183.7939, 27.7782) (183.8358, 27.8294) (183.8567, 27.855) knots 0 0 0 0 0 0 0.01428571 0.02857143 0.04285714 0.05714286 0.07142857 0.08571429 0.1 0.11428571 0.12857143 0.14285714 0.15714286 0.17142857 0.18571429 0.2 0.21428571 0.22857143 0.24285714 0.25714286 0.27142857 0.28571429 0.3 0.31428571 0.32857143 0.34285714 0.35714286 0.37142857 0.38571429 0.4 0.41428571 0.42857143 0.44285714 0.45714286 0.47142857 0.48571429 0.5 0.51428571 0.52857143 0.54285714 0.55714286 0.57142857 0.58571429 0.6 0.61428571 0.62857143 0.64285714 0.65714286 0.67142857 0.68571429 0.7 0.71428571 0.72857143 0.74285714 0.75714286 0.77142857 0.78571429 0.8 0.81428571 0.82857143 0.84285714 0.85714286 0.87142857 0.88571429 0.9 0.91428571 0.92857143 0.94285714 0.95714286 0.97142857 0.98571429 1 1 1 1 1 1
  arc A59 (183.8567, 27.855) -> (182.2139, 31.821) centre (111, 0) ccw
  spline S29 degree 5 poles (182.2139, 31.821) (182.181, 31.8243) (182.1152, 31.8309) (182.0164, 31.8406) (181.8848, 31.853) (181.7205, 31.8678) (181.5563, 31.8819) (181.3921, 31.8952) (181.2281, 31.9078) (181.0642, 31.9197) (180.9005, 31.9308) (180.7368, 31.9412) (180.5733, 31.9508) (180.41, 31.9597) (180.2468, 31.9678) (180.0837, 31.9751) (179.9208, 31.9817) (179.758, 31.9875) (179.5954, 31.9925) (179.4329, 31.9967) (179.2706, 32.0002) (179.1085, 32.0028) (178.9465, 32.0047) (178.7847, 32.0057) (178.6231, 32.006) (178.4617, 32.0054) (178.3004, 32.004) (178.1394, 32.0017) (177.9785, 31.9987) (177.8179, 31.9948) (177.6575, 31.99) (177.4972, 31.9844) (177.3372, 31.9779) (177.1775, 31.9705) (177.0179, 31.9623) (176.8586, 31.9532) (176.6995, 31.9431) (176.5407, 31.9322) (176.3821, 31.9204) (176.2238, 31.9076) (176.0657, 31.8939) (175.908, 31.8793) (175.7505, 31.8637) (175.5933, 31.847) (175.4364, 31.8294) (175.2798, 31.8108) (175.1236, 31.7913) (174.9676, 31.7707) (174.8119, 31.7491) (174.6566, 31.7265) (174.5017, 31.7027) (174.3471, 31.6778) (174.193, 31.6517) (174.0393, 31.6244) (173.886, 31.5959) (173.7331, 31.5662) (173.5806, 31.5355) (173.4284, 31.5037) (173.2767, 31.4708) (173.1255, 31.4366) (172.9748, 31.4009) (172.8248, 31.3633) (172.6756, 31.3239) (172.5272, 31.2825) (172.3795, 31.2394) (172.2323, 31.1951) (172.0854, 31.1498) (171.939, 31.1036) (171.7931, 31.0562) (171.6483, 31.0063) (171.5053, 30.9525) (171.3928, 30.905) (171.3097, 30.8664) (171.255, 30.8393) (171.2278, 30.8254) knots -1 -1 -1 -1 -1 -1 -0.98571429 -0.97142857 -0.95714286 -0.94285714 -0.92857143 -0.91428571 -0.9 -0.88571429 -0.87142857 -0.85714286 -0.84285714 -0.82857143 -0.81428571 -0.8 -0.78571429 -0.77142857 -0.75714286 -0.74285714 -0.72857143 -0.71428571 -0.7 -0.68571429 -0.67142857 -0.65714286 -0.64285714 -0.62857143 -0.61428571 -0.6 -0.58571429 -0.57142857 -0.55714286 -0.54285714 -0.52857143 -0.51428571 -0.5 -0.48571429 -0.47142857 -0.45714286 -0.44285714 -0.42857143 -0.41428571 -0.4 -0.38571429 -0.37142857 -0.35714286 -0.34285714 -0.32857143 -0.31428571 -0.3 -0.28571429 -0.27142857 -0.25714286 -0.24285714 -0.22857143 -0.21428571 -0.2 -0.18571429 -0.17142857 -0.15714286 -0.14285714 -0.12857143 -0.11428571 -0.1 -0.08571429 -0.07142857 -0.05714286 -0.04285714 -0.02857143 -0.01428571 0 0 0 0 0 0
  line L29 (171.2278, 30.8254) -> (170.6672, 30.5385)
  arc A60 (168.0036, 31.3549) -> (170.6672, 30.5385) centre (169.756, 32.3188) ccw
  arc A61 (168.0036, 31.3549) -> (166.656, 33.6891) centre (111, 0) ccw
  arc A62 (167.2807, 36.4041) -> (166.656, 33.6891) centre (168.3669, 34.7248) ccw
  line L30 (167.2807, 36.4041) -> (167.8094, 36.7461)
  spline S30 degree 5 poles (167.8094, 36.7461) (167.8351, 36.7627) (167.886, 36.7965) (167.9609, 36.8491) (168.0583, 36.9229) (168.1764, 37.0198) (168.292, 37.1203) (168.406, 37.2229) (168.5192, 37.3266) (168.6318, 37.4312) (168.7438, 37.5365) (168.855, 37.6429) (168.9651, 37.7507) (169.0739, 37.8602) (169.1813, 37.9713) (169.2876, 38.0839) (169.3929, 38.1978) (169.4972, 38.3128) (169.6008, 38.4286) (169.7037, 38.5454) (169.8058, 38.6629) (169.9072, 38.7814) (170.0077, 38.9009) (170.1074, 39.0213) (170.2062, 39.1427) (170.3042, 39.265) (170.4015, 39.3882) (170.498, 39.5122) (170.5938, 39.637) (170.6889, 39.7625) (170.7833, 39.8889) (170.877, 40.0159) (170.97, 40.1437) (171.0623, 40.2723) (171.1538, 40.4016) (171.2447, 40.5316) (171.3349, 40.6624) (171.4245, 40.7938) (171.5133, 40.9259) (171.6015, 41.0586) (171.6891, 41.192) (171.776, 41.3261) (171.8623, 41.4608) (171.9479, 41.5961) (172.0329, 41.7321) (172.1172, 41.8686) (172.2009, 42.0058) (172.284, 42.1435) (172.3665, 42.2819) (172.4483, 42.4208) (172.5295, 42.5603) (172.6101, 42.7004) (172.6901, 42.841) (172.7695, 42.9822) (172.8483, 43.124) (172.9264, 43.2662) (173.004, 43.4091) (173.081, 43.5524) (173.1573, 43.6963) (173.2331, 43.8407) (173.3083, 43.9856) (173.3829, 44.131) (173.4569, 44.2769) (173.5303, 44.4233) (173.6031, 44.5702) (173.6754, 44.7176) (173.747, 44.8654) (173.8181, 45.0138) (173.8886, 45.1626) (173.9586, 45.3118) (174.0279, 45.4616) (174.0829, 45.5817) (174.124, 45.6721) (174.1512, 45.7324) (174.1648, 45.7626) knots 0 0 0 0 0 0 0.01428571 0.02857143 0.04285714 0.05714286 0.07142857 0.08571429 0.1 0.11428571 0.12857143 0.14285714 0.15714286 0.17142857 0.18571429 0.2 0.21428571 0.22857143 0.24285714 0.25714286 0.27142857 0.28571429 0.3 0.31428571 0.32857143 0.34285714 0.35714286 0.37142857 0.38571429 0.4 0.41428571 0.42857143 0.44285714 0.45714286 0.47142857 0.48571429 0.5 0.51428571 0.52857143 0.54285714 0.55714286 0.57142857 0.58571429 0.6 0.61428571 0.62857143 0.64285714 0.65714286 0.67142857 0.68571429 0.7 0.71428571 0.72857143 0.74285714 0.75714286 0.77142857 0.78571429 0.8 0.81428571 0.82857143 0.84285714 0.85714286 0.87142857 0.88571429 0.9 0.91428571 0.92857143 0.94285714 0.95714286 0.97142857 0.98571429 1 1 1 1 1 1
  arc A63 (174.1648, 45.7626) -> (171.5515, 49.1682) centre (111, 0) ccw
  spline S31 degree 5 poles (171.5515, 49.1682) (171.5188, 49.1629) (171.4535, 49.1523) (171.3557, 49.136) (171.2253, 49.114) (171.0628, 49.0857) (170.9005, 49.0568) (170.7385, 49.0272) (170.5768, 48.997) (170.4154, 48.966) (170.2544, 48.9344) (170.0936, 48.902) (169.9332, 48.869) (169.7731, 48.8353) (169.6134, 48.8009) (169.4539, 48.7658) (169.2949, 48.73) (169.1361, 48.6934) (168.9778, 48.6562) (168.8197, 48.6182) (168.6621, 48.5795) (168.5048, 48.5401) (168.3478, 48.5) (168.1913, 48.4591) (168.0351, 48.4175) (167.8794, 48.3752) (167.724, 48.3321) (167.569, 48.2883) (167.4144, 48.2437) (167.2603, 48.1983) (167.1065, 48.1522) (166.9532, 48.1053) (166.8004, 48.0576) (166.6479, 48.0091) (166.496, 47.9599) (166.3444, 47.9098) (166.1934, 47.859) (166.0428, 47.8073) (165.8927, 47.7549) (165.743, 47.7016) (165.5939, 47.6474) (165.4453, 47.5924) (165.2972, 47.5366) (165.1497, 47.4799) (165.0027, 47.4222) (164.8563, 47.3638) (164.7104, 47.3044) (164.5651, 47.2442) (164.4203, 47.183) (164.2762, 47.121) (164.1326, 47.0579) (163.9898, 46.9939) (163.8477, 46.9288) (163.7063, 46.8626) (163.5656, 46.7954) (163.4256, 46.7271) (163.2862, 46.658) (163.1475, 46.5879) (163.0094, 46.5169) (162.8722, 46.4447) (162.7359, 46.3712) (162.6008, 46.2961) (162.4669, 46.2194) (162.3342, 46.141) (162.2027, 46.0611) (162.072, 45.9802) (161.9418, 45.8985) (161.8123, 45.816) (161.6837, 45.7324) (161.5567, 45.6467) (161.4325, 45.5577) (161.3361, 45.4828) (161.2659, 45.424) (161.2201, 45.3836) (161.1974, 45.3631) knots -1 -1 -1 -1 -1 -1 -0.98571429 -0.97142857 -0.95714286 -0.94285714 -0.92857143 -0.91428571 -0.9 -0.88571429 -0.87142857 -0.85714286 -0.84285714 -0.82857143 -0.81428571 -0.8 -0.78571429 -0.77142857 -0.75714286 -0.74285714 -0.72857143 -0.71428571 -0.7 -0.68571429 -0.67142857 -0.65714286 -0.64285714 -0.62857143 -0.61428571 -0.6 -0.58571429 -0.57142857 -0.55714286 -0.54285714 -0.52857143 -0.51428571 -0.5 -0.48571429 -0.47142857 -0.45714286 -0.44285714 -0.42857143 -0.41428571 -0.4 -0.38571429 -0.37142857 -0.35714286 -0.34285714 -0.32857143 -0.31428571 -0.3 -0.28571429 -0.27142857 -0.25714286 -0.24285714 -0.22857143 -0.21428571 -0.2 -0.18571429 -0.17142857 -0.15714286 -0.14285714 -0.12857143 -0.11428571 -0.1 -0.08571429 -0.07142857 -0.05714286 -0.04285714 -0.02857143 -0.01428571 0 0 0 0 0 0
  line L31 (161.1974, 45.3631) -> (160.7302, 44.9409)
  arc A64 (157.946, 45.0401) -> (160.7302, 44.9409) centre (159.3892, 46.4248) ccw
  arc A65 (157.946, 45.0401) -> (156.0401, 46.946) centre (111, 0) ccw
  arc A66 (155.9409, 49.7302) -> (156.0401, 46.946) centre (157.4248, 48.3892) ccw
  line L32 (155.9409, 49.7302) -> (156.3631, 50.1974)
  spline S32 degree 5 poles (156.3631, 50.1974) (156.3836, 50.2201) (156.424, 50.2659) (156.4828, 50.3361) (156.5577, 50.4325) (156.6467, 50.5567) (156.7324, 50.6837) (156.816, 50.8123) (156.8985, 50.9418) (156.9802, 51.072) (157.0611, 51.2027) (157.141, 51.3342) (157.2194, 51.4669) (157.2961, 51.6008) (157.3712, 51.7359) (157.4447, 51.8722) (157.5169, 52.0094) (157.5879, 52.1475) (157.658, 52.2862) (157.7271, 52.4256) (157.7954, 52.5656) (157.8626, 52.7063) (157.9288, 52.8477) (157.9939, 52.9898) (158.0579, 53.1326) (158.121, 53.2762) (158.183, 53.4203) (158.2442, 53.5651) (158.3044, 53.7104) (158.3638, 53.8563) (158.4222, 54.0027) (158.4799, 54.1497) (158.5366, 54.2972) (158.5924, 54.4453) (158.6474, 54.5939) (158.7016, 54.743) (158.7549, 54.8927) (158.8073, 55.0428) (158.859, 55.1934) (158.9098, 55.3444) (158.9599, 55.496) (159.0091, 55.6479) (159.0576, 55.8004) (159.1053, 55.9532) (159.1522, 56.1065) (159.1983, 56.2603) (159.2437, 56.4144) (159.2883, 56.569) (159.3321, 56.724) (159.3752, 56.8794) (159.4175, 57.0351) (159.4591, 57.1913) (159.5, 57.3478) (159.5401, 57.5048) (159.5795, 57.6621) (159.6182, 57.8197) (159.6562, 57.9778) (159.6934, 58.1361) (159.73, 58.2949) (159.7658, 58.4539) (159.8009, 58.6134) (159.8353, 58.7731) (159.869, 58.9332) (159.902, 59.0936) (159.9344, 59.2544) (159.966, 59.4154) (159.997, 59.5768) (160.0272, 59.7385) (160.0568, 59.9005) (160.0857, 60.0628) (160.114, 60.2253) (160.136, 60.3557) (160.1523, 60.4535) (160.1629, 60.5188) (160.1682, 60.5515) knots 0 0 0 0 0 0 0.01428571 0.02857143 0.04285714 0.05714286 0.07142857 0.08571429 0.1 0.11428571 0.12857143 0.14285714 0.15714286 0.17142857 0.18571429 0.2 0.21428571 0.22857143 0.24285714 0.25714286 0.27142857 0.28571429 0.3 0.31428571 0.32857143 0.34285714 0.35714286 0.37142857 0.38571429 0.4 0.41428571 0.42857143 0.44285714 0.45714286 0.47142857 0.48571429 0.5 0.51428571 0.52857143 0.54285714 0.55714286 0.57142857 0.58571429 0.6 0.61428571 0.62857143 0.64285714 0.65714286 0.67142857 0.68571429 0.7 0.71428571 0.72857143 0.74285714 0.75714286 0.77142857 0.78571429 0.8 0.81428571 0.82857143 0.84285714 0.85714286 0.87142857 0.88571429 0.9 0.91428571 0.92857143 0.94285714 0.95714286 0.97142857 0.98571429 1 1 1 1 1 1
  arc A67 (160.1682, 60.5515) -> (156.7626, 63.1648) centre (111, 0) ccw
  spline S33 degree 5 poles (156.7626, 63.1648) (156.7324, 63.1512) (156.6721, 63.124) (156.5817, 63.0829) (156.4616, 63.0279) (156.3118, 62.9586) (156.1626, 62.8886) (156.0138, 62.8181) (155.8654, 62.747) (155.7176, 62.6754) (155.5702, 62.6031) (155.4233, 62.5303) (155.2769, 62.4569) (155.131, 62.3829) (154.9856, 62.3083) (154.8407, 62.2331) (154.6963, 62.1573) (154.5524, 62.081) (154.4091, 62.004) (154.2662, 61.9264) (154.124, 61.8483) (153.9822, 61.7695) (153.841, 61.6901) (153.7004, 61.6101) (153.5603, 61.5295) (153.4208, 61.4483) (153.2819, 61.3665) (153.1435, 61.284) (153.0058, 61.2009) (152.8686, 61.1172) (152.7321, 61.0329) (152.5961, 60.9479) (152.4608, 60.8623) (152.3261, 60.776) (152.192, 60.6891) (152.0586, 60.6015) (151.9259, 60.5133) (151.7938, 60.4245) (151.6624, 60.3349) (151.5316, 60.2447) (151.4016, 60.1538) (151.2723, 60.0623) (151.1437, 59.97) (151.0159, 59.877) (150.8889, 59.7833) (150.7625, 59.6889) (150.637, 59.5938) (150.5122, 59.498) (150.3882, 59.4015) (150.265, 59.3042) (150.1427, 59.2062) (150.0213, 59.1074) (149.9009, 59.0077) (149.7814, 58.9072) (149.6629, 58.8058) (149.5454, 58.7037) (149.4286, 58.6008) (149.3128, 58.4972) (149.1978, 58.3929) (149.0839, 58.2876) (148.9713, 58.1813) (148.8602, 58.0739) (148.7507, 57.9651) (148.6429, 57.855) (148.5365, 57.7438) (148.4312, 57.6318) (148.3266, 57.5192) (148.2229, 57.406) (148.1203, 57.292) (148.0198, 57.1764) (147.9229, 57.0583) (147.8491, 56.9609) (147.7965, 56.886) (147.7627, 56.8351) (147.7461, 56.8094) knots -1 -1 -1 -1 -1 -1 -0.98571429 -0.97142857 -0.95714286 -0.94285714 -0.92857143 -0.91428571 -0.9 -0.88571429 -0.87142857 -0.85714286 -0.84285714 -0.82857143 -0.81428571 -0.8 -0.78571429 -0.77142857 -0.75714286 -0.74285714 -0.72857143 -0.71428571 -0.7 -0.68571429 -0.67142857 -0.65714286 -0.64285714 -0.62857143 -0.61428571 -0.6 -0.58571429 -0.57142857 -0.55714286 -0.54285714 -0.52857143 -0.51428571 -0.5 -0.48571429 -0.47142857 -0.45714286 -0.44285714 -0.42857143 -0.41428571 -0.4 -0.38571429 -0.37142857 -0.35714286 -0.34285714 -0.32857143 -0.31428571 -0.3 -0.28571429 -0.27142857 -0.25714286 -0.24285714 -0.22857143 -0.21428571 -0.2 -0.18571429 -0.17142857 -0.15714286 -0.14285714 -0.12857143 -0.11428571 -0.1 -0.08571429 -0.07142857 -0.05714286 -0.04285714 -0.02857143 -0.01428571 0 0 0 0 0 0
  line L33 (147.7461, 56.8094) -> (147.4041, 56.2807)
  arc A68 (144.6891, 55.656) -> (147.4041, 56.2807) centre (145.7248, 57.3669) ccw
  arc A69 (144.6891, 55.656) -> (142.3549, 57.0036) centre (111, 0) ccw
  arc A70 (141.5385, 59.6672) -> (142.3549, 57.0036) centre (143.3188, 58.756) ccw
  line L34 (141.5385, 59.6672) -> (141.8254, 60.2278)